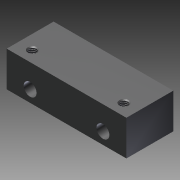
# Autodesk Inventor part: MG5-5-ap
Saved by Autodesk Inventor 2011 SP1 (Build 150282100, 282)
## iProperties
Created: 2015-02-01
Part Number: MG5-5-ap
Catalog Web Link: www.cadenas.de
Description: HMEN, HMER-attachment plate-Latch Magnets for Plate
Vendor: MISUMI
Document SubType Name: Modeling
Designer: psAdmin
Manufacturer: MISUMI
Mass: 14.1005 g
Surface Area: 50.1144 cm^2
Volume: 14.1005 cm^3
Density: 1 g/cm^3
Category: PARTsolutions
Company: MISUMI
Title: MG5-5-ap
Author: Cadenas PARTsolutions
Comments: Latch Magnets for Plate
PSOL_IDENT_0: {\\10.0.0.236\data_v8\23d-libs\misumi\metric\39_accessories_for_al_extrusions\hmen_attachment_plate.
PSOL_IDENT_1: prj},179 {VTYP=3D},{NB=MG5-5-ap},{LINA=MG5-5-ap},{NN=HMEN, HMER-attachment plate},{DATE=17.11.2014 0
PSOL_IDENT_2: 5:31:11},{GEOMDATE=07.06.2009 15:48:00},{VERSION=},{LINEID=10},{LINESUBID=-1},{WBVAR=}  {NB=MG5-5-ap
PSOL_IDENT_3: },{LINA=MG5-5-ap},{KT=DUMMY},{PN=MG5-5},{TYPE=MG},{MAT=6063 Aluminum Alloy},{NO=5-5},{MG=1},{AP=MG5-
PSOL_IDENT_4: 5},{APP=1},{M=4.000},{A=51.000},{B=20.000},{H=0.000},{L=0.000},{T=15.000},{G=31.000},{S=6.000},{V=5.
PSOL_IDENT_5: 000},{Y=10.000},{E=0.000},{X=15.000},{F=0.000},{MMIN=3.242},{X1=0},{P1=7.5},{PX=19.5},{PY=5},{XY=0.0
PSOL_IDENT_6: 00},{YY=15.000},{P11=0.0}
SUPPLIER: MISUMI
ARTICLENO: MG5-5-ap
BOMINFO: MG5-5-ap
CREATOR: CADENAS GmbH
Autodesk Inventor part; units mm, degrees
sketch "Sketch_14" plane through (0, 0, 0) normal (0, 1, 0) x (-1, 0, 0)
  line L0 (25.5, 7.5) -> (-25.5, 7.5)
  line L1 (-25.5, 7.5) -> (-25.5, -7.5)
  line L2 (-25.5, -7.5) -> (25.5, -7.5)
  line L3 (25.5, -7.5) -> (25.5, 7.5)
  circle A0 centre (-15.5, -2.5) radius 2.75
  circle A1 centre (15.5, -2.5) radius 2.75
  constraints: 8 end point, 2 centre point
extrude "Extrusion1" add sketch "Sketch_14" along normal mid plane 20
sketch "Sketch_2" plane through (19.5, 0, 0) normal (1, 0, 0) x (0, 0, -1)
  line L0 (7.5, -5) -> (-7.5, -5)
  line L1 (-7.5, -5) -> (-7.5, -3)
  line L2 (-7.5, -3) -> (-7.121, -3.379)
  line L3 (-7.121, -3.379) -> (7.121, -3.379)
  line L4 (7.121, -3.379) -> (7.5, -3)
  line L5 (7.5, -3) -> (7.5, -5)
  line L6 (7.5, -5) -> (-7.5, -5)
  constraints: 14 end point
revolve "Revolution1" cut sketch "Sketch_2" angle 360 about axis through (19.5, -5, -7.5) along (0, 0, -1)
thread "Thread1" size "M4x0.7" class "6H" standard "ISO Metric profile" full length
sketch "Sketch_3" plane through (-19.5, 0, 0) normal (1, 0, 0) x (0, 0, -1)
  line L0 (7.5, -5) -> (-7.5, -5)
  line L1 (-7.5, -5) -> (-7.5, -3)
  line L2 (-7.5, -3) -> (-7.121, -3.379)
  line L3 (-7.121, -3.379) -> (7.121, -3.379)
  line L4 (7.121, -3.379) -> (7.5, -3)
  line L5 (7.5, -3) -> (7.5, -5)
  line L6 (7.5, -5) -> (-7.5, -5)
  constraints: 14 end point
revolve "Revolution2" cut sketch "Sketch_3" angle 360 about axis through (-19.5, -5, -7.5) along (0, 0, -1)
thread "Thread2" size "M4x0.7" class "6H" standard "ISO Metric profile" full length
ref_plane "att_plate_magnet_XY" through (19.5, -5, 7.5) normal (0, 0, 1) x (1, 0, 0)
ref_plane "att_plate_magnet_YZ" through (19.5, -5, 7.5) normal (1, 0, 0) x (0, 1, 0)
ref_plane "att_plate_magnet_ZX" through (19.5, -5, 7.5) normal (0, 1, 0) x (0, 0, 1)
ref_plane "to_magnetT_XY" through (-19.5, -5, 7.5) normal (0, 0, 1) x (1, 0, 0)
ref_plane "to_magnetT_YZ" through (-19.5, -5, 7.5) normal (1, 0, 0) x (0, 1, 0)
ref_plane "to_magnetT_ZX" through (-19.5, -5, 7.5) normal (0, 1, 0) x (0, 0, 1)
ref_plane "c1_XY" through (-15.5, 10, -2.5) normal (0, 1, 0) x (1, 0, 0)
ref_plane "c1_YZ" through (-15.5, 10, -2.5) normal (1, 0, 0) x (0, 0, -1)
ref_plane "c1_ZX" through (-15.5, 10, -2.5) normal (0, 0, -1) x (0, 1, 0)
ref_plane "c2_XY" through (15.5, 10, -2.5) normal (0, 1, 0) x (1, 0, 0)
ref_plane "c2_YZ" through (15.5, 10, -2.5) normal (1, 0, 0) x (0, 0, -1)
ref_plane "c2_ZX" through (15.5, 10, -2.5) normal (0, 0, -1) x (0, 1, 0)
ref_plane "c3_XY" through (-15.5, -10, -2.5) normal (0, 1, 0) x (1, 0, 0)
ref_plane "c3_YZ" through (-15.5, -10, -2.5) normal (1, 0, 0) x (0, 0, -1)
ref_plane "c3_ZX" through (-15.5, -10, -2.5) normal (0, 0, -1) x (0, 1, 0)
ref_plane "c4_XY" through (15.5, -10, -2.5) normal (0, 1, 0) x (1, 0, 0)
ref_plane "c4_YZ" through (15.5, -10, -2.5) normal (1, 0, 0) x (0, 0, -1)
ref_plane "c4_ZX" through (15.5, -10, -2.5) normal (0, 0, -1) x (0, 1, 0)
ref_plane "cc3_XY" through (-15.5, 10, -2.5) normal (0, 1, 0) x (1, 0, 0)
ref_plane "cc3_YZ" through (-15.5, 10, -2.5) normal (1, 0, 0) x (0, 0, -1)
ref_plane "cc3_ZX" through (-15.5, 10, -2.5) normal (0, 0, -1) x (0, 1, 0)
ref_plane "cc4_XY" through (15.5, 10, -2.5) normal (0, 1, 0) x (1, 0, 0)
ref_plane "cc4_YZ" through (15.5, 10, -2.5) normal (1, 0, 0) x (0, 0, -1)
ref_plane "cc4_ZX" through (15.5, 10, -2.5) normal (0, 0, -1) x (0, 1, 0)
ref_plane "cc1_XY" through (-15.5, -10, -2.5) normal (0, 1, 0) x (1, 0, 0)
ref_plane "cc1_YZ" through (-15.5, -10, -2.5) normal (1, 0, 0) x (0, 0, -1)
ref_plane "cc1_ZX" through (-15.5, -10, -2.5) normal (0, 0, -1) x (0, 1, 0)
ref_plane "cc2_XY" through (15.5, -10, -2.5) normal (0, 1, 0) x (1, 0, 0)
ref_plane "cc2_YZ" through (15.5, -10, -2.5) normal (1, 0, 0) x (0, 0, -1)
ref_plane "cc2_ZX" through (15.5, -10, -2.5) normal (0, 0, -1) x (0, 1, 0)
ref_plane "d1_XY" through (15.5, 15, -5) normal (0, 1, 0) x (1, 0, 0)
ref_plane "d1_YZ" through (15.5, 15, -5) normal (1, 0, 0) x (0, 0, -1)
ref_plane "d1_ZX" through (15.5, 15, -5) normal (0, 0, -1) x (0, 1, 0)
ref_plane "d2_XY" through (-15.5, 15, -5) normal (0, 1, 0) x (1, 0, 0)
ref_plane "d2_YZ" through (-15.5, 15, -5) normal (1, 0, 0) x (0, 0, -1)
ref_plane "d2_ZX" through (-15.5, 15, -5) normal (0, 0, -1) x (0, 1, 0)
ref_plane "e1_XY" through (-15.5, 15, -5) normal (0, 1, 0) x (1, 0, 0)
ref_plane "e1_YZ" through (-15.5, 15, -5) normal (1, 0, 0) x (0, 0, -1)
ref_plane "e1_ZX" through (-15.5, 15, -5) normal (0, 0, -1) x (0, 1, 0)
ref_plane "e2_XY" through (15.5, 15, -5) normal (0, 1, 0) x (1, 0, 0)
ref_plane "e2_YZ" through (15.5, 15, -5) normal (1, 0, 0) x (0, 0, -1)
ref_plane "e2_ZX" through (15.5, 15, -5) normal (0, 0, -1) x (0, 1, 0)
ref_plane "p1_XY" through (15.5, 10, 0) normal (0, 1, 0) x (1, 0, 0)
ref_plane "p1_YZ" through (15.5, 10, 0) normal (1, 0, 0) x (0, 0, -1)
ref_plane "p1_ZX" through (15.5, 10, 0) normal (0, 0, -1) x (0, 1, 0)
ref_plane "p2_XY" through (-15.5, 10, 0) normal (0, 1, 0) x (1, 0, 0)
ref_plane "p2_YZ" through (-15.5, 10, 0) normal (1, 0, 0) x (0, 0, -1)
ref_plane "p2_ZX" through (-15.5, 10, 0) normal (0, 0, -1) x (0, 1, 0)
ref_plane "xxxx_XY" through (0, 0, 0) normal (0, 0, 1) x (1, 0, 0)
ref_plane "xxxx_YZ" through (0, 0, 0) normal (1, 0, 0) x (0, 1, 0)
ref_plane "xxxx_ZX" through (0, 0, 0) normal (0, 1, 0) x (0, 0, 1)
ref_plane "p11_XY" through (15.5, 10, 31) normal (0, 1, 0) x (1, 0, 0)
ref_plane "p11_YZ" through (15.5, 10, 31) normal (1, 0, 0) x (0, 0, -1)
ref_plane "p11_ZX" through (15.5, 10, 31) normal (0, 0, -1) x (0, 1, 0)
ref_plane "p22_XY" through (-15.5, 10, 31) normal (0, 1, 0) x (1, 0, 0)
ref_plane "p22_YZ" through (-15.5, 10, 31) normal (1, 0, 0) x (0, 0, -1)
ref_plane "p22_ZX" through (-15.5, 10, 31) normal (0, 0, -1) x (0, 1, 0)
ref_plane "plate_to_magnet_XY" through (-19.5, -5, 7.5) normal (0, 1, 0) x (1, 0, 0)
ref_plane "plate_to_magnet_YZ" through (-19.5, -5, 7.5) normal (1, 0, 0) x (0, 0, -1)
ref_plane "plate_to_magnet_ZX" through (-19.5, -5, 7.5) normal (0, 0, -1) x (0, 1, 0)
body "Solid1"
